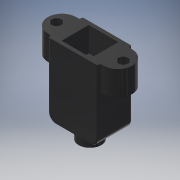
# Autodesk Inventor part: panel-mount
Saved by Autodesk Inventor 2017 (Build 210142000, 142)
## iProperties
Created: 2020-10-05
Part Number: panel-mount
Material: Generic
Document SubType Name: Modeling
Designer: Joe Ferner
Density: 1 g/cm^3
Appearance: Default
Author: Joe Ferner
Autodesk Inventor part; units mm, degrees
ref_plane "YZ Plane" through (0, 0, 0) normal (1, 0, 0) x (0, 1, 0)
ref_plane "XZ Plane" through (0, 0, 0) normal (0, 1, 0) x (-1, 0, 0)
ref_plane "XY Plane" through (0, 0, 0) normal (0, 0, 1) x (1, 0, 0)
sketch "Sketch1" plane through (0, 0, 0) normal (0, 0, 1) x (1, 0, 0)
  line L0 (0.5, 0) -> (19.5, 0)
  line L1 (19.5, 14) -> (0.5, 14)
  line L2 (-0.5, 12.795) -> (-1.405, 12.795)
  line L3 (-1.405, 1.205) -> (-0.5, 1.205)
  line L4 (20.5, 12.795) -> (21.405, 12.795)
  line L5 (21.405, 1.205) -> (20.5, 1.205)
  line L6 (0, 13.5) -> (0, 13.295)
  line L7 (0, 0.705) -> (0, 0.5)
  line L8 (20, 0.5) -> (20, 0.705)
  line L9 (20, 13.295) -> (20, 13.5)
  circle A0 centre (-3.6, 7) radius 2
  circle A1 centre (23.6, 7) radius 2
  line L10 (3.975, 12.525) -> (16.025, 12.525)
  line L11 (16.025, 12.525) -> (16.025, 1.475)
  line L12 (16.025, 1.475) -> (3.975, 1.475)
  line L13 (3.975, 1.475) -> (3.975, 12.525)
  arc A2 (0.5, 14) -> (0, 13.5) centre (0.5, 13.5) ccw
  arc A3 (-0.5, 12.795) -> (0, 13.295) centre (-0.5, 13.295) ccw
  arc A4 (20, 13.5) -> (19.5, 14) centre (19.5, 13.5) ccw
  arc A5 (20, 13.295) -> (20.5, 12.795) centre (20.5, 13.295) ccw
  arc A6 (20.5, 1.205) -> (20, 0.705) centre (20.5, 0.705) ccw
  arc A7 (19.5, 0) -> (20, 0.5) centre (19.5, 0.5) ccw
  arc A8 (0, 0.5) -> (0.5, 0) centre (0.5, 0.5) ccw
  arc A9 (0, 0.705) -> (-0.5, 1.205) centre (-0.5, 0.705) ccw
  line L14 (10, 15.3107) -> (10, 19.4603)
  arc A10 (-1.405, 12.795) -> (-1.405, 1.205) centre (-1.405, 7) ccw
  arc A11 (21.405, 1.205) -> (21.405, 12.795) centre (21.405, 7) ccw
  line L15 (-7.2, 7) -> (-7.2, 15.3107)
  point P0 (0, 0)
  point P1 (20, 14)
  point P2 (20, 0)
  point P3 (0, 14)
  point P4 (0, 12.795)
  point P5 (0, 1.205)
  point P6 (20, 12.795)
  point P7 (20, 1.205)
  dimension "d0" = 11.59
  dimension "d1" = 1.205
  dimension "d2" = 4
  dimension "width" = 20
  dimension "height" = 14
  dimension "d7" = 12.05
  dimension "d8" = 11.05
  dimension "d9" = 3.975
  dimension "d10" = 1.475
  dimension "d13" = 0.5
  dimension "d31" = 27.2
  dimension "d32" = 13.6
  dimension "d33" = 10
  dimension "d34" = 34.4
  dimension "d35" = 17.2
  constraints: 32 end point, 21 point on circle, 20 tangent, 18 point on line, 12 centre point, 9 parallel, 8 equal radius, 4 horizontal, 3 perpendicular, 2 collinear, 2 horizontal alignment, 2 vertical, 2 vertical alignment
  measures "d0" distance between parallel lines of L2 L3
  measures "d1" distance between parallel lines of L0 L3
  measures "d2" diameter of A0
  measures "width" distance of point (0, 0) point (20, 0)
  measures "height" distance between parallel lines of L1 L0
  measures "d7" distance of L11.end L12.end
  measures "d8" distance of L10.end L11.end
  measures "d9" distance between parallel lines of L7 L13
  measures "d10" distance between parallel lines of L0 L12
  measures "d13" radius of A2
  measures "d31" distance of A1.centre A0.centre
  measures "d32" distance from line of L14 A0.centre
  measures "d33" distance from line of L6.end L14
  measures "d35" distance between parallel lines of L14 L15
extrude "Extrusion1" add sketch "Sketch1" against normal blind 10
sketch "Sketch3" plane through (0, 0, -10) normal (0, 0, -1) x (-1, 0, 0)
  line L0 (-19.5, 14) -> (-0.5, 14)
  line L1 (0, 13.5) -> (0, 0.5)
  line L2 (-0.5, 0) -> (-19.5, 0)
  line L3 (-20, 0.5) -> (-20, 13.5)
  line L4 (-0.5, 0) -> (-19.5, 0) projected
  line L5 (0, 0.5) -> (0, 0.705) projected
  arc A0 (0, 13.5) -> (-0.5, 14) centre (-0.5, 13.5) ccw
  arc A1 (-0.5, 0) -> (0, 0.5) centre (-0.5, 0.5) ccw
  arc A2 (-20, 0.5) -> (-19.5, 0) centre (-19.5, 0.5) ccw
  arc A3 (-19.5, 14) -> (-20, 13.5) centre (-19.5, 13.5) ccw
  point P0 (0, 0)
  point P1 (-20, 14)
  point P2 (0, 0)
  point P3 (0, 14)
  point P4 (-20, 0)
  dimension "d14" = 20
  dimension "d15" = 14
  dimension "d16" = 0
  dimension "d17" = 0
  dimension "d20" = 0.5
  constraints: 8 end point, 8 point on circle, 8 point on line, 8 tangent, 4 centre point, 3 equal radius, 2 parallel, 1 horizontal, 1 perpendicular
  measures "d14" distance of point (0, 0) point (-20, 0)
  measures "d15" distance of point (0, 14) point (0, 0)
  measures "d16" distance between parallel lines of L4 L2
  measures "d17" distance between parallel lines of L5 L1
  measures "d20" radius of A0
extrude "Extrusion2" add sketch "Sketch3" along normal blind 19.32
sketch "Sketch6" plane through (0.5, 14, 0) normal (0, 1, 0) x (1, 0, 0)
  line L0 (-0.5, 0) -> (-0.5, 29.32) projected
  line L1 (-0.5, 29.32) -> (-0.5, 26.32)
  line L2 (-0.5, 29.32) -> (2.5, 29.32)
  arc A0 (2.5, 29.32) -> (-0.5, 26.32) centre (2.5, 26.32) ccw
  line L3 (19.5, 0) -> (19.5, 29.32) projected
  line L4 (19.5, 29.32) -> (19.5, 26.32)
  line L5 (19.5, 29.32) -> (16.5, 29.32)
  line L6 (0, 29.32) -> (19, 29.32) projected
  arc A1 (19.5, 26.32) -> (16.5, 29.32) centre (16.5, 26.32) ccw
  dimension "d36" = 3
  constraints: 8 end point, 4 point on circle, 4 tangent, 3 point on line, 2 centre point, 1 horizontal, 1 horizontal alignment
  measures "d36" radius of A0
extrude "Extrusion4" cut sketch "Sketch6" against normal through all
fillet "Fillet2" radius 0.5 10 edges at (18.4186, 14, -28.9634) (19.8751, 13.8307, -27.1768) (1.5814, 14, -28.9634) (0.1247, 13.8304, -27.176) (10, 14, -29.32) (1.5814, 0, -28.9634) (0.1249, 0.1694, -27.1767) (18.4186, 0, -28.9634) (19.8753, 0.1696, -27.176) (10, 0, -29.32)
sketch "Sketch7" plane through (0, 0, -29.32) normal (0, 0, -1) x (-1, 0, 0)
  circle A0 centre (-10, 7) radius 4.625
  line L0 (-3, 14) -> (-17, 14) projected
  line L1 (-20, 0.5) -> (-20, 13.5) projected
  point P0 (0, 0)
  dimension "d40" = 9.25
  dimension "d41" = 7
  dimension "d42" = 10
  constraints: 1 centre point
  measures "d40" diameter of A0
  measures "d41" distance from line of L0 A0.centre
  measures "d42" distance from line of L1 A0.centre
extrude "Extrusion5" add sketch "Sketch7" along normal blind 5
equation "\"d1\" = -0.5 * d0 + 0.5 * height"
equation "\"d9\" = -0.5 * d7 + 0.5 * width"
equation "\"d10\" = -0.5 * d8 + 0.5 * height"
equation "\"d32\" = 0.5 * d31"
equation "\"d33\" = 0.5 * width"
equation "\"d35\" = 0.5 * d34"
equation "\"d16\" = -0.5 * d15 + 0.5 * height"
equation "\"d17\" = -0.5 * d14 + 0.5 * width"
equation "\"d41\" = 0.5 * height"
equation "\"d42\" = 0.5 * width"
body "Solid1"
